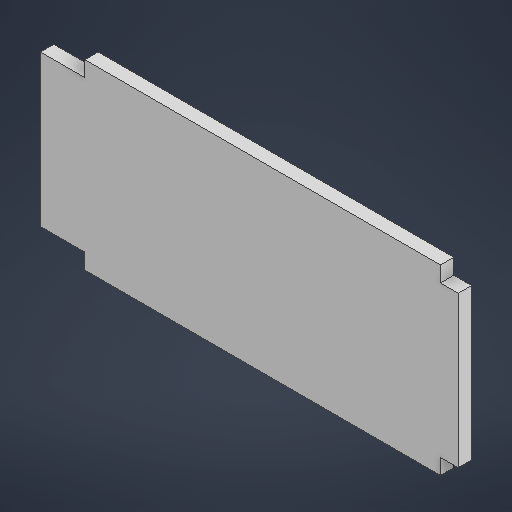
# Autodesk Inventor part: Battary_holder_part2
Saved by Autodesk Inventor 2027 (Build 310192000, 192)
## iProperties
Created: 2026-05-15
Part Number: Battary_holder_part2
Material: Generic
Document SubType Name: Modeling
Designer: alexy
Density: 1 g/cm^3
Appearance: Default
Author: alexy
Autodesk Inventor part; units mm, degrees
ref_plane "YZ Plane" through (0, 0, 0) normal (1, 0, 0) x (0, 1, 0)
ref_plane "XZ Plane" through (0, 0, 0) normal (0, 1, 0) x (-1, 0, 0)
ref_plane "XY Plane" through (0, 0, 0) normal (0, 0, 1) x (1, 0, 0)
sketch "Sketch1" plane through (0, 0, 0) normal (0, 0, 1) x (1, 0, 0)
  line L0 (0, 0) -> (80, 0)
  line L1 (80, 0) -> (80, 41)
  line L2 (80, 41) -> (0, 41)
  line L3 (0, 41) -> (0, 0)
  line L4 (84, 37.5) -> (80, 37.5)
  line L5 (80, 37.5) -> (80, 3.5)
  line L6 (80, 3.5) -> (84, 3.5)
  line L7 (84, 3.5) -> (84, 37.5)
  line L8 (84, 37.5) -> (80, 3.5) construction
  line L9 (80, 37.5) -> (84, 3.5) construction
  line L10 (-10, 37.5) -> (0, 37.5)
  line L11 (0, 37.5) -> (0, 3.5)
  line L12 (0, 3.5) -> (-10, 3.5)
  line L13 (-10, 3.5) -> (-10, 37.5)
  line L14 (-10, 37.5) -> (0, 3.5) construction
  line L15 (0, 37.5) -> (-10, 3.5) construction
  point P0 (82, 20.5)
  point P1 (-5, 20.5)
  point P2 (0, 37.5)
  point P3 (0, 37.5)
  point P4 (80, 37.5)
  point P5 (110, 40)
  point P6 (0, 40)
  point P7 (80, 20.5)
  dimension "d0" = 10
  dimension "d1" = 4
  dimension "d2" = 80
  dimension "d3" = 41
  dimension "d4" = 34
  constraints: 32 end point, 6 parallel, 5 midpoint, 3 horizontal, 3 horizontal alignment, 3 perpendicular, 3 point on line
  measures "d0" distance of L10.start L10.end
  measures "d1" distance of L4.start L4.end
  measures "d2" distance of L0.start L0.end
  measures "d3" distance of L0.end L1.end
  measures "d4" distance of L6.end L4.start
extrude "Extrusion1" add sketch "Sketch1" along normal blind 3
body "Solid1"
